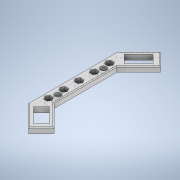
# Autodesk Inventor part: Side_Frame
Saved by Autodesk Inventor 2021 (Build 250183000, 183)
## iProperties
Created: 2021-08-13
Part Number: Side_Frame
Material: Generic
Document SubType Name: Modeling
Designer: rbnsmathew
Density: 1 g/cm^3
Appearance: Default
Author: rbnsmathew
Autodesk Inventor part; units mm, degrees
ref_plane "YZ Plane" through (0, 0, 0) normal (1, 0, 0) x (0, 1, 0)
ref_plane "XZ Plane" through (0, 0, 0) normal (0, 1, 0) x (-1, 0, 0)
ref_plane "XY Plane" through (0, 0, 0) normal (0, 0, 1) x (1, 0, 0)
sketch "Sketch1" plane through (0, 0, 0) normal (0, 1, 0) x (-1, 0, 0)
  line L0 (0, 0) -> (-29.0466, 0)
  line L1 (0, 58.5031) -> (-5.7395, 64.2426)
  line L2 (6.2813, 43.0294) -> (-10.3357, 59.6464)
  line L3 (-10.3357, 59.6464) -> (-1.1433, 68.8388)
  line L4 (-1.1433, 68.8388) -> (15.4737, 52.2218)
  line L5 (15.4737, 52.2218) -> (6.2813, 43.0294)
  line L6 (6.2813, 43.0294) -> (-1.1433, 68.8388) construction
  line L7 (-10.3357, 59.6464) -> (15.4737, 52.2218) construction
  line L8 (7.802, 36.0648) -> (-17.3003, 61.1671)
  line L9 (-17.3003, 61.1671) -> (-2.664, 75.8034)
  line L10 (-2.664, 75.8034) -> (22.4383, 50.7011)
  line L11 (22.4383, 50.7011) -> (7.802, 36.0648)
  line L12 (7.802, 36.0648) -> (-2.664, 75.8034) construction
  line L13 (-17.3003, 61.1671) -> (22.4383, 50.7011) construction
  line L14 (7.802, 36.0648) -> (7.802, -0.7306)
  line L15 (22.4383, 50.7011) -> (22.4383, -0.4008)
  line L16 (6.2813, -43.0294) -> (-10.3357, -59.6464)
  line L17 (-10.3357, -59.6464) -> (-1.1433, -68.8388)
  line L18 (-1.1433, -68.8388) -> (15.4737, -52.2218)
  line L19 (15.4737, -52.2218) -> (6.2813, -43.0294)
  line L20 (-10.3357, -59.6464) -> (15.4737, -52.2218) construction
  line L21 (7.802, -36.0648) -> (-17.3003, -61.1671)
  line L22 (-17.3003, -61.1671) -> (-2.664, -75.8034)
  line L23 (-2.664, -75.8034) -> (22.4383, -50.7011)
  line L24 (22.4383, -50.7011) -> (7.802, -36.0648)
  line L25 (7.802, -36.0648) -> (-2.664, -75.8034) construction
  line L26 (7.802, -36.0648) -> (7.802, -0.7306)
  line L27 (22.4383, -50.7011) -> (22.4383, -0.4008)
  point P0 (2.569, 55.9341)
  point P1 (-1.4969, 60)
  dimension "d0" = 45
  dimension "d1" = 6
  dimension "d2" = 23.5
  dimension "d3" = 13
  dimension "d4" = 60
  dimension "d6" = 6
  constraints: 56 end point, 8 symmetric about line, 5 midpoint, 5 parallel, 4 vertical, 2 perpendicular, 2 point on line, 1 horizontal
  measures "d0" angle of L0 L1
  measures "d1" distance from line of L3 point (-1.497, 60)
  measures "d2" distance between parallel lines of L3 L5
  measures "d3" distance between parallel lines of L4 L2
  measures "d4" distance from line of L0 point (-1.497, 60)
  measures "d6" distance between parallel lines of L9 L3
extrude "Extrusion1" add sketch "Sketch1" along normal blind 6
sketch "Sketch3" plane through (0, 0, 0) normal (0, -1, 0) x (1, 0, 0)
  line L0 (-9.3663, 0) -> (-22.4383, 0)
  line L1 (-22.4383, -50.7011) -> (-22.4383, 50.7011) projected
  circle A0 centre (-15.2967, -35) radius 3.75
  circle A1 centre (-15.2967, 0) radius 3.75
  circle A2 centre (-15.2967, -17.5) radius 3.75
  circle A3 centre (-15.2967, 35) radius 3.75
  line L2 (-19.0467, -35) -> (-17.1717, -31.7524)
  line L3 (-17.1717, -31.7524) -> (-13.4217, -31.7524)
  line L4 (-13.4217, -31.7524) -> (-11.5467, -35)
  line L5 (-11.5467, -35) -> (-13.4217, -38.2476)
  line L6 (-13.4217, -38.2476) -> (-17.1717, -38.2476)
  line L7 (-17.1717, -38.2476) -> (-19.0467, -35)
  line L8 (-19.0467, -17.5) -> (-17.1717, -14.2524)
  line L9 (-17.1717, -14.2524) -> (-13.4217, -14.2524)
  line L10 (-13.4217, -14.2524) -> (-11.5467, -17.5)
  line L11 (-11.5467, -17.5) -> (-13.4217, -20.7476)
  line L12 (-13.4217, -20.7476) -> (-17.1717, -20.7476)
  line L13 (-17.1717, -20.7476) -> (-19.0467, -17.5)
  line L14 (-19.0467, 0) -> (-17.1717, 3.2476)
  line L15 (-17.1717, 3.2476) -> (-13.4217, 3.2476)
  line L16 (-13.4217, 3.2476) -> (-11.5467, 0)
  line L17 (-11.5467, 0) -> (-13.4217, -3.2476)
  line L18 (-13.4217, -3.2476) -> (-17.1717, -3.2476)
  line L19 (-17.1717, -3.2476) -> (-19.0467, 0)
  line L20 (-19.0467, 35) -> (-17.1717, 38.2476)
  line L21 (-17.1717, 38.2476) -> (-13.4217, 38.2476)
  line L22 (-13.4217, 38.2476) -> (-11.5467, 35)
  line L23 (-11.5467, 35) -> (-13.4217, 31.7524)
  line L24 (-13.4217, 31.7524) -> (-17.1717, 31.7524)
  line L25 (-17.1717, 31.7524) -> (-19.0467, 35)
  circle A4 centre (-15.2967, 17.5) radius 3.75
  line L26 (-19.0467, 17.5) -> (-17.1717, 20.7476)
  line L27 (-17.1717, 20.7476) -> (-13.4217, 20.7476)
  line L28 (-13.4217, 20.7476) -> (-11.5467, 17.5)
  line L29 (-11.5467, 17.5) -> (-13.4217, 14.2524)
  line L30 (-13.4217, 14.2524) -> (-17.1717, 14.2524)
  line L31 (-17.1717, 14.2524) -> (-19.0467, 17.5)
  point P0 (0, 0)
  dimension "d15" = 7.5
  dimension "d16" = 7.5
  dimension "d17" = 7.5
  dimension "d19" = 7.5
  dimension "d20" = 7.5
  constraints: 62 end point, 6 coincident, 5 horizontal alignment, 1 midpoint, 1 point on line, 75 other
extrude "Extrusion3" cut sketch "Sketch3" against normal blind 6 contours L17 L18 L19 L0 | L0 L14 L15 L16 | L5 L6 L7 L2 L3 L4 | L11 L12 L13 L8 L9 L10 | L23 L24 L25 L20 L21 L22 | L29 L30 L31 L26 L27 L28
sketch "Sketch5" plane through (0, 6, 0) normal (0, 1, 0) x (1, 0, 0)
  line L0 (-17.1717, -3.2476) -> (-19.0467, 0) projected
  line L1 (-19.0467, 0) -> (-17.1717, 3.2476) projected
  line L2 (-17.1717, 3.2476) -> (-13.4217, 3.2476) projected
  line L3 (-13.4217, 3.2476) -> (-11.5467, 0) projected
  line L4 (-11.5467, 0) -> (-13.4217, -3.2476) projected
  line L5 (-13.4217, -3.2476) -> (-17.1717, -3.2476) projected
  line L6 (-13.4217, 20.7476) -> (-11.5467, 17.5) projected
  line L7 (-11.5467, 17.5) -> (-13.4217, 14.2524) projected
  line L8 (-13.4217, 14.2524) -> (-17.1717, 14.2524) projected
  line L9 (-17.1717, 14.2524) -> (-19.0467, 17.5) projected
  line L10 (-19.0467, 17.5) -> (-17.1717, 20.7476) projected
  line L11 (-17.1717, 20.7476) -> (-13.4217, 20.7476) projected
  line L12 (-13.4217, -31.7524) -> (-11.5467, -35) projected
  line L13 (-11.5467, -35) -> (-13.4217, -38.2476) projected
  line L14 (-13.4217, -38.2476) -> (-17.1717, -38.2476) projected
  line L15 (-17.1717, -38.2476) -> (-19.0467, -35) projected
  line L16 (-19.0467, -35) -> (-17.1717, -31.7524) projected
  line L17 (-17.1717, -31.7524) -> (-13.4217, -31.7524) projected
  line L18 (-13.4217, 38.2476) -> (-11.5467, 35) projected
  line L19 (-11.5467, 35) -> (-13.4217, 31.7524) projected
  line L20 (-13.4217, 31.7524) -> (-17.1717, 31.7524) projected
  line L21 (-17.1717, 31.7524) -> (-19.0467, 35) projected
  line L22 (-19.0467, 35) -> (-17.1717, 38.2476) projected
  line L23 (-17.1717, 38.2476) -> (-13.4217, 38.2476) projected
  line L24 (-13.4217, -14.2524) -> (-11.5467, -17.5) projected
  line L25 (-11.5467, -17.5) -> (-13.4217, -20.7476) projected
  line L26 (-13.4217, -20.7476) -> (-17.1717, -20.7476) projected
  line L27 (-17.1717, -20.7476) -> (-19.0467, -17.5) projected
  line L28 (-19.0467, -17.5) -> (-17.1717, -14.2524) projected
  line L29 (-17.1717, -14.2524) -> (-13.4217, -14.2524) projected
  line L30 (-7.802, -36.0648) -> (-7.802, 36.0648) projected
  line L31 (-7.802, 36.0648) -> (17.3003, 61.1671) projected
  line L32 (17.3003, 61.1671) -> (2.664, 75.8034) projected
  line L33 (2.664, 75.8034) -> (-22.4383, 50.7011) projected
  line L34 (-22.4383, 50.7011) -> (-22.4383, -50.7011) projected
  line L35 (-22.4383, -50.7011) -> (2.664, -75.8034) projected
  line L36 (2.664, -75.8034) -> (17.3003, -61.1671) projected
  line L37 (17.3003, -61.1671) -> (-7.802, -36.0648) projected
  line L38 (1.1433, 68.8388) -> (10.3357, 59.6464) projected
  line L39 (10.3357, 59.6464) -> (-6.2813, 43.0294) projected
  line L40 (-6.2813, 43.0294) -> (-15.4737, 52.2218) projected
  line L41 (-15.4737, 52.2218) -> (1.1433, 68.8388) projected
  line L42 (1.1433, -68.8388) -> (-15.4737, -52.2218) projected
  line L43 (-15.4737, -52.2218) -> (-6.2813, -43.0294) projected
  line L44 (-6.2813, -43.0294) -> (10.3357, -59.6464) projected
  line L45 (10.3357, -59.6464) -> (1.1433, -68.8388) projected
  line L46 (-13.4217, -31.7524) -> (-11.5467, -35) projected
  line L47 (-11.5467, -35) -> (-7.802, -35)
  line L48 (-7.802, -36.0648) -> (-7.802, 36.0648) projected
  line L49 (-11.5467, -17.5) -> (-7.802, -17.5)
  line L50 (-11.5467, 17.5) -> (-7.802, 17.5)
  line L51 (-13.4217, 31.7524) -> (-11.5467, 35) projected
  line L52 (-11.5467, 35) -> (-7.802, 35)
  line L53 (-7.802, -26.25) -> (-16.5311, -26.25)
  line L54 (-7.802, 26.25) -> (-17.8697, 26.25)
  circle A0 centre (-13.302, -26.25) radius 2.05
  circle A1 centre (-13.302, 26.25) radius 2.05
  point P0 (0, 0)
  dimension "d34" = 8.75
  dimension "d35" = 8.75
  dimension "d38" = 4.1
  dimension "d39" = 5.5
  dimension "d40" = 4.1
  dimension "d41" = 5.5
  constraints: 12 end point, 8 point on line, 3 perpendicular, 2 centre point, 2 horizontal, 1 parallel
  measures "d34" distance between parallel lines of L54 L50
  measures "d35" distance between parallel lines of L53 L47
  measures "d38" diameter of A0
  measures "d39" distance of A0.centre L53.start
  measures "d40" diameter of A1
  measures "d41" distance of A1.centre L54.start
extrude "Extrusion4" cut sketch "Sketch5" against normal blind 10 contours A1 L54 | L54 A1 | A0 L53 | L53 A0
chamfer "Chamfer1" distance 1 angle 45 8 edges at (-7.802, 6, 0) (-22.4383, 6, 0) (4.7492, 6, 48.616) (9.9822, 6, 68.4853) (-9.8871, 6, 63.2523) (4.7492, 6, -48.616) (-9.8871, 6, -63.2523) (9.9822, 6, -68.4853)
chamfer "Chamfer2" distance 0.5 angle 45 30 edges at (-15.2967, 6, 3.2476) (-18.1092, 6, 1.6238) (-18.1092, 6, -1.6238) (-15.2967, 6, -3.2476) (-12.4842, 6, -1.6238) (-12.4842, 6, 1.6238) (-15.2967, 6, -14.2524) (-18.1092, 6, -15.8762) (-18.1092, 6, -19.1238) (-15.2967, 6, -20.7476) (-12.4842, 6, -19.1238) (-12.4842, 6, -15.8762) (-18.1092, 6, -33.3762) (-18.1092, 6, -36.6238) (-15.2967, 6, -38.2476) (-12.4842, 6, -36.6238) (-12.4842, 6, -33.3762) (-15.2967, 6, -31.7524) (-15.2967, 6, 14.2524) (-18.1092, 6, 15.8762) (-18.1092, 6, 19.1238) (-15.2967, 6, 20.7476) (-12.4842, 6, 19.1238) (-12.4842, 6, 15.8762) (-15.2967, 6, 31.7524) (-18.1092, 6, 33.3762) (-18.1092, 6, 36.6238) (-15.2967, 6, 38.2476) (-12.4842, 6, 36.6238) (-12.4842, 6, 33.3762)
sketch "Sketch6" plane through (0, 6, 0) normal (0, 1, 0) x (1, 0, 0)
  circle A0 centre (-13.302, -26.25) radius 2.05 projected
  circle A1 centre (-13.302, -26.25) radius 3.5
  circle A2 centre (-13.302, 26.25) radius 2.05 projected
  circle A3 centre (-13.302, 26.25) radius 3.5
  point P0 (0, 0)
  dimension "d50" = 7
  dimension "d51" = 7
  constraints: 2 centre point, 2 coincident
  measures "d50" diameter of A1
  measures "d51" diameter of A3
extrude "Extrusion5" cut sketch "Sketch6" against normal blind 3
equation "\"d15\" = d17"
equation "\"d16\" = d17"
equation "\"d19\" = d17"
equation "\"d20\" = d17"
equation "\"d51\" = d50"
body "Solid1"
